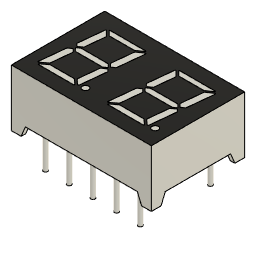
DICE_2281 (Autodesk Fusion 360 design; units mm, degrees)
Autodesk Fusion 360 part; units mm, degrees
note: some values were not read from the file. Set by a fixed rule: which sketch regions a step uses.
sketch "Footprint" plane through (0, 0, 0) normal (0, 0, 1) x (1, 0, 0)
  line L0 (-7.5, 5) -> (7.5, 5)
  line L1 (7.5, 5) -> (7.5, -5)
  line L2 (7.5, -5) -> (-7.5, -5)
  line L3 (-7.5, -5) -> (-7.5, 5)
  line L4 (-7.5, 5) -> (7.5, -5) construction
  line L5 (7.5, 5) -> (-7.5, -5) construction
  dimension "d1" = 15
  dimension "d2" = 10
  constraint horizontal L0
  constraint perpendicular L0 L1
  constraint parallel L0 L2
  constraint parallel L1 L3
  constraint coincident L4 origin
  constraint coincident L5 origin
  measures "d1" distance of L1.end L2.end
  measures "d2" distance of L0.end L1.end
extrude "Extrude Height" add sketch "Footprint" along normal blind 5 makes body 1
sketch "Bottom Feature Profile" plane through (0, 0, 0) normal (0, 0, -1) x (1, 0, 0)
  line L0 (7.5, 5) -> (-7.5, 5)
  line L1 (-7.5, 5) -> (-7.5, -5)
  line L2 (-7.5, -5) -> (7.5, -5)
  line L3 (7.5, -5) -> (7.5, 5)
  circle A0 centre (-5.08, -3.76) radius 0.225
  circle A1 centre (-2.54, -3.76) radius 0.225
  circle A2 centre (0, -3.76) radius 0.225
  circle A3 centre (2.54, -3.76) radius 0.225
  circle A4 centre (5.08, -3.76) radius 0.225
  circle A5 centre (-5.08, 3.76) radius 0.225
  circle A6 centre (-2.54, 3.76) radius 0.225
  circle A7 centre (0, 3.76) radius 0.225
  circle A8 centre (2.54, 3.76) radius 0.225
  circle A9 centre (5.08, 3.76) radius 0.225
  line L4 (-5.08, 3.76) -> (5.08, -3.76) construction
  line L5 (-7.5, 5) -> (-7, 5)
  line L6 (-7, 5) -> (-7, 3.5)
  line L7 (-7, 3.5) -> (-7.5, 3.5)
  line L8 (-7.5, 3.5) -> (-7.5, 5)
  line L9 (-7.5, 5) -> (-6, 5)
  line L10 (-6, 5) -> (-6, 4.5)
  line L11 (-6, 4.5) -> (-7.5, 4.5)
  line L12 (-7.5, 4.5) -> (-7.5, 5)
  dimension "d5" = 0.45
  dimension "d8" = 2.54
  dimension "d9" = 7.52
  dimension "d12" = 0.5
  dimension "d13" = 1.5
  dimension "d14" = 1.5
  dimension "d15" = 0.5
  constraint coincident A5.centre L4.start
  constraint midpoint origin L4
  constraint horizontal L5
  constraint vertical L6
  constraint horizontal L7
  constraint vertical L8
  constraint coincident L0.end L1.start
  constraint horizontal L9
  constraint vertical L10
  constraint horizontal L11
  constraint vertical L12
  constraint coincident A4.centre L4.end
  measures "d5" diameter of A0
  measures "d12" distance of L0.end L5.end
  measures "d13" distance of L0.end L7.end
  measures "d14" distance of L0.end L9.end
  measures "d15" distance of L0.end L11.end
extrude "Extrude Pins" add sketch "Bottom Feature Profile" along normal blind 5 contours A0 | A1 | A2 | A3 | A4 | A5 | A6 | A7 | A8 | A9 bodies 1
extrude "Extrude Foot" add sketch "Bottom Feature Profile" along normal blind 1.1 separate body contours L0 L6 L9 L10 L11 | L0 L1 L5 L6 L8 L9 L11 L12 | L1 L6 L7 L8 L11 makes body 2
sketch "Foot Cut Y" plane through (0, -5, 0) normal (0, -1, 0) x (1, 0, 0)
  line L0 (-7.5, 0) -> (7.5, 0)
  line L1 (7.5, 0) -> (7.5, 5)
  line L2 (7.5, 5) -> (-7.5, 5)
  line L3 (-7.5, 5) -> (-7.5, 0)
  line L4 (-7.5, 0) -> (-10.0594, 0) construction
  line L5 (-6, -1.1) -> (-7.5, -1.1)
  line L6 (-6, 0) -> (-6.4556, -1.1)
  line L7 (-6, 0) -> (-8.5594, 0) construction
  line L8 (-6.4556, -1.1) -> (-6, -1.1)
  line L9 (-6, -1.1) -> (-6, 0)
  point P0 (-6, 0)
  dimension "d24" = 112.5
  constraint horizontal L4
  constraint coincident L0.start L3.end
  constraint horizontal L7
  constraint coincident P0 L6.start
  constraint coincident L5 L6.end
  constraint coincident L5.start L8.end
  measures "d24" angle of L6 L7
extrude "Foot Cut Y (1)" cut sketch "Foot Cut Y" against normal blind 0.5 contours L5 L6 L8 L9 bodies 2
sketch "Foot Cut X" plane through (-7.5, 0, 0) normal (-1, 0, 0) x (0, -1, 0)
  line L0 (5, 0) -> (5, 5)
  line L1 (5, 5) -> (-5, 5)
  line L2 (-5, 5) -> (-5, 0)
  line L3 (-5, 0) -> (5, 0)
  line L4 (5, -1.1) -> (3.5, -1.1)
  line L5 (5, 0) -> (6.1906, 0) construction
  line L6 (3.5, 0) -> (3.9556, -1.1)
  line L7 (3.5, 0) -> (4.6906, 0) construction
  line L8 (3.9556, -1.1) -> (3.5, -1.1)
  line L9 (3.5, -1.1) -> (3.5, 0)
  point P0 (3.5, 0)
  dimension "d25" = 67.5
  constraint horizontal L5
  constraint coincident L0.start L3.end
  constraint horizontal L7
  constraint coincident P0 L6.start
  constraint coincident L4 L6.end
  constraint coincident L4.end L8.end
  measures "d25" angle of L6 L7
extrude "Foot Cut X (1)" cut sketch "Foot Cut X" against normal blind 0.5 contours L4 L6 L8 L9 bodies 2
mirror "Mirror1" about plane through (0, 0, 0) normal (1, 0, 0) of bodies 2 makes body 3
mirror "Mirror2" about plane through (0, 0, 0) normal (0, 1, 0) of bodies 2 3 makes body 4 at (-7.5, 4.1519, -0.3667) makes body 5 at (7.5, 4.1519, -0.3667)
combine "Combine1" operation add target body 1 tool bodies 2 3 4 5
sketch "Characters" plane through (0, 0, 5) normal (0, 0, 1) x (-1, 0, 0)
  line L0 (7.5, -4.5932) -> (7.5, 4.5932)
  line L1 (7.5, 4.5932) -> (-7.5, 4.5932)
  line L2 (-7.5, 4.5932) -> (-7.5, -4.5932)
  line L3 (-7.5, -4.5932) -> (7.5, -4.5932)
  ellipse E0 centre (1.3951, 3.1591) end of major axis (1.0528, 3.1591) minor radius 0.3426 (1.0528, 3.1595) -> (1.7373, 3.1595) cw
  ellipse E1 centre (1.3951, 3.1599) end of major axis (1.0528, 3.1599) minor radius 0.3426 (1.7373, 3.1595) -> (1.0528, 3.1595) cw
  line L4 (5.4663, 2.893) -> (2.8577, 2.893)
  line L5 (2.8577, 2.893) -> (2.2553, 3.4413)
  line L6 (2.2553, 3.4413) -> (2.3282, 3.5021)
  line L7 (2.3282, 3.5021) -> (6.1163, 3.5021)
  line L8 (6.1163, 3.5021) -> (6.1866, 3.4435)
  line L9 (6.1866, 3.4435) -> (5.4663, 2.893)
  line L10 (1.5906, -3.502) -> (1.5434, -3.4552)
  line L11 (1.5434, -3.4552) -> (2.2677, -2.9484)
  line L12 (2.2677, -2.9484) -> (4.9629, -2.9484)
  line L13 (4.9629, -2.9484) -> (5.4728, -3.4552)
  line L14 (5.4728, -3.4552) -> (5.4058, -3.502)
  line L15 (5.4058, -3.502) -> (1.5906, -3.502)
  line L16 (6.3481, 3.3087) -> (6.4068, 3.2598)
  line L17 (6.4068, 3.2598) -> (6.1108, 0.4384)
  line L18 (6.1108, 0.4384) -> (5.7152, 0.1616)
  line L19 (5.7152, 0.1616) -> (5.3833, 0.4915)
  line L20 (5.3833, 0.4915) -> (5.6205, 2.7527)
  line L21 (5.6205, 2.7527) -> (6.3481, 3.3087)
  line L22 (1.6274, -0.3717) -> (1.9944, -0.1149)
  line L23 (1.9944, -0.1149) -> (2.3503, -0.4686)
  line L24 (2.3503, -0.4686) -> (2.1042, -2.8143)
  line L25 (2.1042, -2.8143) -> (1.3967, -3.3094)
  line L26 (1.3967, -3.3094) -> (1.3265, -3.2396)
  line L27 (1.3265, -3.2396) -> (1.6274, -0.3717)
  line L28 (2.4545, 0.525) -> (1.975, 0.1894)
  line L29 (1.975, 0.1894) -> (1.7135, 0.4492)
  line L30 (1.7135, 0.4492) -> (2.0055, 3.2329)
  line L31 (2.0055, 3.2329) -> (2.0938, 3.3065)
  line L32 (2.0938, 3.3065) -> (2.6894, 2.7644)
  line L33 (2.6894, 2.7644) -> (2.4545, 0.525)
  line L34 (5.6927, -0.0529) -> (5.3331, -0.3045)
  line L35 (5.3331, -0.3045) -> (2.4236, -0.3045)
  line L36 (2.4236, -0.3045) -> (2.064, 0.0529)
  line L37 (2.064, 0.0529) -> (2.4236, 0.3046)
  line L38 (2.4236, 0.3046) -> (5.3331, 0.3046)
  line L39 (5.3331, 0.3046) -> (5.6927, -0.0529)
  line L40 (5.2746, -0.5442) -> (5.719, -0.2333)
  line L41 (5.719, -0.2333) -> (6.01, -0.5225)
  line L42 (6.01, -0.5225) -> (5.7205, -3.2819)
  line L43 (5.7205, -3.2819) -> (5.6476, -3.3329)
  line L44 (5.6476, -3.3329) -> (5.0449, -2.7339)
  line L45 (5.0449, -2.7339) -> (5.2746, -0.5442)
  ellipse E2 centre (-6.0645, 3.1592) end of major axis (-6.4068, 3.1592) minor radius 0.3426 (-6.4068, 3.1595) -> (-5.7223, 3.1595) cw
  ellipse E3 centre (-6.0645, 3.1598) end of major axis (-6.4068, 3.1598) minor radius 0.3426 (-5.7223, 3.1595) -> (-6.4068, 3.1595) cw
  line L46 (-1.9933, 2.893) -> (-4.6019, 2.893)
  line L47 (-4.6019, 2.893) -> (-5.2043, 3.4413)
  line L48 (-5.2043, 3.4413) -> (-5.1313, 3.5021)
  line L49 (-5.1313, 3.5021) -> (-1.3433, 3.5021)
  line L50 (-1.3433, 3.5021) -> (-1.273, 3.4435)
  line L51 (-1.273, 3.4435) -> (-1.9933, 2.893)
  line L52 (-5.869, -3.502) -> (-5.9161, -3.4552)
  line L53 (-5.9161, -3.4552) -> (-5.1919, -2.9484)
  line L54 (-5.1919, -2.9484) -> (-2.4967, -2.9484)
  line L55 (-2.4967, -2.9484) -> (-1.9868, -3.4552)
  line L56 (-1.9868, -3.4552) -> (-2.0537, -3.502)
  line L57 (-2.0537, -3.502) -> (-5.869, -3.502)
  line L58 (-1.1115, 3.3087) -> (-1.0528, 3.2598)
  line L59 (-1.0528, 3.2598) -> (-1.3488, 0.4384)
  line L60 (-1.3488, 0.4384) -> (-1.7444, 0.1616)
  line L61 (-1.7444, 0.1616) -> (-2.0763, 0.4915)
  line L62 (-2.0763, 0.4915) -> (-1.8391, 2.7527)
  line L63 (-1.8391, 2.7527) -> (-1.1115, 3.3087)
  line L64 (-5.8322, -0.3717) -> (-5.4652, -0.1149)
  line L65 (-5.4652, -0.1149) -> (-5.1093, -0.4686)
  line L66 (-5.1093, -0.4686) -> (-5.3554, -2.8143)
  line L67 (-5.3554, -2.8143) -> (-6.0628, -3.3094)
  line L68 (-6.0628, -3.3094) -> (-6.1331, -3.2396)
  line L69 (-6.1331, -3.2396) -> (-5.8322, -0.3717)
  line L70 (-5.0051, 0.525) -> (-5.4846, 0.1894)
  line L71 (-5.4846, 0.1894) -> (-5.7461, 0.4492)
  line L72 (-5.7461, 0.4492) -> (-5.4541, 3.2329)
  line L73 (-5.4541, 3.2329) -> (-5.3658, 3.3065)
  line L74 (-5.3658, 3.3065) -> (-4.7702, 2.7644)
  line L75 (-4.7702, 2.7644) -> (-5.0051, 0.525)
  line L76 (-1.7669, -0.0529) -> (-2.1265, -0.3045)
  line L77 (-2.1265, -0.3045) -> (-5.036, -0.3045)
  line L78 (-5.036, -0.3045) -> (-5.3956, 0.0529)
  line L79 (-5.3956, 0.0529) -> (-5.036, 0.3046)
  line L80 (-5.036, 0.3046) -> (-2.1265, 0.3046)
  line L81 (-2.1265, 0.3046) -> (-1.7669, -0.0529)
  line L82 (-2.185, -0.5442) -> (-1.7406, -0.2333)
  line L83 (-1.7406, -0.2333) -> (-1.4496, -0.5225)
  line L84 (-1.4496, -0.5225) -> (-1.7391, -3.2819)
  line L85 (-1.7391, -3.2819) -> (-1.812, -3.3329)
  line L86 (-1.812, -3.3329) -> (-2.4147, -2.7339)
  line L87 (-2.4147, -2.7339) -> (-2.185, -0.5442)
  line L88 (7.5, -4.5932) -> (-7.5, 4.5932) construction
  line L89 (-7.5, -4.5932) -> (7.5, 4.5932) construction
  constraint midpoint L89 origin
extrude "Indent LED" cut sketch "Characters" against normal blind 0.01 contours E0 E1 | L4 L5 L6 L7 L8 L9 | L10 L11 L12 L13 L14 L15 | L16 L17 L18 L19 L20 L21 | L22 L23 L24 L25 L26 L27 | L28 L29 L30 L31 L32 L33 | L34 L35 L36 L37 L38 L39 | L40 L41 L42 L43 L44 L45 | E2 E3 | L46 L47 L48 L49 L50 L51 | L52 L53 L54 L55 L56 L57 | L58 L59 L60 L61 L62 L63 | L64 L65 L66 L67 L68 L69 | L70 L71 L72 L73 L74 L75 | L76 L77 L78 L79 L80 L81 | L82 L83 L84 L85 L86 L87 bodies 1
ref_plane "WorkPlane1" through (-6.9778, -4.4778, -4.2) normal (0, 0, -1) x (-1, 0, 0)
extrude "Trim Leads" cut 10 faces at (-5.1144, -3.6989, -5) (-2.6059, -3.7636, -5) (-0.0134, -3.7014, -5) (2.4741, -3.7636, -5) (5.0456, -3.6989, -5) (-2.6142, 3.7488, -5) (2.4658, 3.7488, -5) (5.135, 3.7935, -5) (-0.0361, 3.8219, -5) (-5.025, 3.7935, -5) along direction (0, 0, -1) up to surface end surface through (-6.9778, -4.4778, -4.2) normal (0, 0, -1) offset 0 on bodies 1 bodies 1
sketch "Pin Origin Reference" plane through (0, 0, -1.1) normal (0, 0, -1) x (1, 0, 0)
  circle A0 centre (-5.08, 3.76) radius 0.225
  point P0 (-5.08, 3.76)
  constraint coincident P0 A0.centre
move_body "Move1" bodies 1 to x (1, 0, 0) y (0, 1, 0) z (0, 0, 1) at (5.08, 3.76, 1.1)
equation "d24 = 90 deg + 22.5 deg"
equation "d25 = 90 deg - 22.5 deg"
equation "segment_d = 0.01 mm" comment "Distance segments are cut into surface"
equation "d32 = -segment_d"
equation "pcb_t = 1.6 mm" comment "PCB thickness (used to trim pins)"
equation "d35 = pcb_t + lead_surplus"
equation "lead_surplus = 1.5 mm" comment "Length the pins extend past the bottom of the PCB"
named bodies: "Dice", "Foot", "Foot (1)", "Foot (2)", "Foot (1) (1)"
